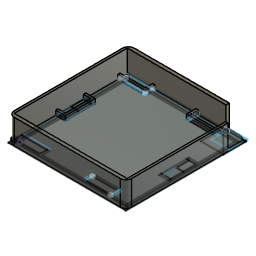
丐17磁悬浮验证底座 (Autodesk Fusion 360 design; units mm, degrees)
Autodesk Fusion 360 part; units mm, degrees
sketch "草图1" plane through (0, 0, 0) normal (0, 1, 0) x (1, 0, 0)
  line L0 (0, 0) -> (95.2, 0)
  line L1 (95.2, 0) -> (95.2, 95.4)
  line L2 (95.2, 95.4) -> (0, 95.4)
  line L3 (0, 95.4) -> (0, 0)
  line L4 (-1.5, 96.9) -> (96.7, 96.9)
  line L5 (96.7, 96.9) -> (96.7, -1.5)
  line L6 (96.7, -1.5) -> (-1.5, -1.5)
  line L7 (-1.5, -1.5) -> (-1.5, 96.9)
  line L8 (-2.5, 97.9) -> (97.7, 97.9)
  line L9 (97.7, 97.9) -> (97.7, -2.5)
  line L10 (97.7, -2.5) -> (-2.5, -2.5)
  line L11 (-2.5, -2.5) -> (-2.5, 97.9)
  line L12 (-4.5, 100.9) -> (99.7, 100.9)
  line L13 (99.7, 100.9) -> (99.7, -5.5)
  line L14 (99.7, -5.5) -> (-4.5, -5.5)
  line L15 (-4.5, -5.5) -> (-4.5, 100.9)
  line L16 (99.7, 100.9) -> (79.7, 100.9)
  line L17 (79.7, 100.9) -> (79.7, 80.9)
  line L18 (79.7, 80.9) -> (99.7, 80.9)
  line L19 (99.7, 80.9) -> (99.7, 100.9)
  line L20 (79.7, 100.9) -> (99.7, 80.9)
  dimension "d1" = 95.2
  dimension "d2" = 95.4
  dimension "d3" = 1.5
  dimension "d4" = 1.5
  dimension "d5" = 1.5
  dimension "d6" = 1.5
  dimension "d7" = 1
  dimension "d8" = 1
  dimension "d9" = 1
  dimension "d10" = 1
  dimension "d11" = 3
  dimension "d12" = 2
  dimension "d13" = 2
  dimension "d14" = 3
  dimension "d21" = 20
  dimension "d22" = 20
  constraint horizontal L0
  constraint vertical L1
  constraint horizontal L2
  constraint vertical L3
  constraint coincident L0.start L3.end
  constraint horizontal L4
  constraint vertical L5
  constraint horizontal L6
  constraint vertical L7
  constraint horizontal L8
  constraint vertical L9
  constraint horizontal L10
  constraint vertical L11
  constraint horizontal L12
  constraint vertical L13
  constraint horizontal L14
  constraint vertical L15
  constraint horizontal L16
  constraint vertical L17
  constraint horizontal L18
  constraint vertical L19
  measures "d1" distance of L0.start L0.end
  measures "d2" distance of L0.start L2.end
  measures "d3" distance of L2 L4
  measures "d4" distance of L1 L5
  measures "d5" distance of L0 L6
  measures "d6" distance of L3 L7
  measures "d7" distance of L4 L8
  measures "d8" distance of L5 L9
  measures "d9" distance of L6 L10
  measures "d10" distance of L7 L11
  measures "d11" distance of L8 L12
  measures "d12" distance of L11 L15
  measures "d13" distance of L9 L13
  measures "d14" distance of L10 L14
  measures "d21" distance of L12.end L16.end
  measures "d22" distance of L12.end L18.end
extrude "拉伸1" add sketch "草图1" along normal blind 2 contours L0 L1 L2 L3 L17 L18 | L0 L1 L2 L3 L4 L5 L6 L7 L17 L18 | L1 L2 L17 L18 L20 | L1 L5 L18 L20 | L2 L4 L17 L20 | L1 L2 L20 | L1 L2 L4 L5 L20 | L4 L5 L6 L7 L8 L9 L10 L11 L17 L18 | L5 L9 L18 L20 | L4 L8 L17 L20 | L4 L5 L8 L9 L20
extrude "拉伸2" add sketch "草图1" along normal blind 22 contours L8 L9 L10 L11 L12 L13 L14 L15 L17 L18 | L9 L18 L20 | L8 L17 L20 | L8 L9 L12 L13 L16 L19 L20
fillet "圆角1" radius 5 4 edges at (-4.5, 11, 5.5) (99.7, 11, 5.5) (-4.5, 11, -100.9) (99.7, 11, -100.9)
extrude "拉伸3" [suppressed]
fillet "圆角2" [suppressed]
sketch "草图2" plane through (0, 2, 0) normal (0, 1, 0) x (-1, 0, 0)
  line L0 (-97.7, -97.9) -> (2.5, -97.9)
  line L1 (2.5, -97.9) -> (2.5, 2.5)
  line L2 (2.5, 2.5) -> (-97.7, 2.5)
  line L3 (-97.7, 2.5) -> (-97.7, -97.9)
  line L4 (2.5, 2.5) -> (2.5, -20)
  line L5 (2.5, -20) -> (-5.5, -20)
  line L6 (-5.5, -20) -> (-5.5, -22)
  line L7 (-5.5, -22) -> (2.5, -22)
  line L8 (2.5, -22) -> (2.5, -20)
  line L9 (-5.5, -20) -> (-3.5, -20)
  line L10 (-3.5, -20) -> (-3.5, 2.5)
  line L11 (-3.5, 2.5) -> (-5.5, 2.5)
  line L12 (-5.5, 2.5) -> (-5.5, -20)
  line L13 (-97.7, 2.5) -> (-91.7, 2.5)
  line L14 (-91.7, 2.5) -> (-91.7, -20)
  line L15 (-91.7, -20) -> (-97.7, -20)
  line L16 (-97.7, -20) -> (-97.7, 2.5)
  line L17 (-97.7, -20) -> (-89.7, -20)
  line L18 (-89.7, -20) -> (-89.7, -23)
  line L19 (-89.7, -23) -> (-97.7, -23)
  line L20 (-97.7, -23) -> (-97.7, -20)
  line L21 (-89.7, -20) -> (-91.7, -20)
  line L22 (-91.7, -20) -> (-91.7, 2.5)
  line L23 (-91.7, 2.5) -> (-89.7, 2.5)
  line L24 (-89.7, 2.5) -> (-89.7, -20)
  line L25 (-91.7, -97.9) -> (-91.7, -75.4)
  line L26 (-91.7, -97.9) -> (-97.7, -97.9)
  line L27 (-97.7, -97.9) -> (-97.7, -75.4)
  line L28 (-97.7, -75.4) -> (-91.7, -75.4)
  line L29 (2.5, -97.9) -> (2.5, -75.4)
  line L30 (-3.5, -75.4) -> (2.5, -75.4)
  line L31 (-3.5, -97.9) -> (-3.5, -75.4)
  line L32 (2.5, -97.9) -> (-3.5, -97.9)
  line L33 (2.5, -75.4) -> (-5.5, -75.4)
  line L34 (-5.5, -75.4) -> (-5.5, -73.4)
  line L35 (-5.5, -73.4) -> (2.5, -73.4)
  line L36 (2.5, -73.4) -> (2.5, -75.4)
  line L37 (-5.5, -75.4) -> (-3.5, -75.4)
  line L38 (-3.5, -75.4) -> (-3.5, -97.9)
  line L39 (-3.5, -97.9) -> (-5.5, -97.9)
  line L40 (-5.5, -97.9) -> (-5.5, -75.4)
  line L41 (-97.7, -75.4) -> (-89.7, -75.4)
  line L42 (-89.7, -75.4) -> (-89.7, -73.4)
  line L43 (-89.7, -73.4) -> (-97.7, -73.4)
  line L44 (-97.7, -73.4) -> (-97.7, -75.4)
  line L45 (-89.7, -75.4) -> (-91.7, -75.4)
  line L46 (-91.7, -75.4) -> (-91.7, -97.9)
  line L47 (-91.7, -97.9) -> (-89.7, -97.9)
  line L48 (-89.7, -97.9) -> (-89.7, -75.4)
  line L49 (-47.6, -97.9) -> (-47.6, -91.9)
  line L50 (-47.6, -91.9) -> (-36.35, -91.9)
  line L51 (-47.6, -91.9) -> (-58.85, -91.9)
  line L52 (-36.35, -91.9) -> (-58.85, -91.9)
  line L53 (-58.85, -91.9) -> (-58.85, -97.9)
  line L54 (-58.85, -97.9) -> (-36.35, -97.9)
  line L55 (-36.35, -97.9) -> (-36.35, -91.9)
  line L56 (-47.6, 2.5) -> (-36.35, 2.5)
  line L57 (-36.35, -3.5) -> (-36.35, 2.5)
  line L58 (-58.85, -3.5) -> (-36.35, -3.5)
  line L59 (-36.35, 2.5) -> (-58.85, 2.5)
  line L60 (-58.85, 2.5) -> (-58.85, -3.5)
  line L61 (-36.35, -97.9) -> (-34.35, -97.9)
  line L62 (-34.35, -97.9) -> (-34.35, -89.9)
  line L63 (-34.35, -89.9) -> (-36.35, -89.9)
  line L64 (-36.35, -89.9) -> (-36.35, -97.9)
  line L65 (-36.35, -89.9) -> (-58.85, -89.9)
  line L66 (-58.85, -89.9) -> (-58.85, -91.9)
  line L67 (-58.85, -91.9) -> (-36.35, -91.9)
  line L68 (-36.35, -91.9) -> (-36.35, -89.9)
  line L69 (-58.85, -89.9) -> (-60.85, -89.9)
  line L70 (-60.85, -89.9) -> (-60.85, -97.9)
  line L71 (-60.85, -97.9) -> (-58.85, -97.9)
  line L72 (-58.85, -97.9) -> (-58.85, -89.9)
  line L73 (-36.35, 2.5) -> (-34.35, 2.5)
  line L74 (-34.35, 2.5) -> (-34.35, -5.5)
  line L75 (-34.35, -5.5) -> (-36.35, -5.5)
  line L76 (-36.35, -5.5) -> (-36.35, 2.5)
  line L77 (-58.85, 2.5) -> (-60.85, 2.5)
  line L78 (-60.85, 2.5) -> (-60.85, -5.5)
  line L79 (-60.85, -5.5) -> (-58.85, -5.5)
  line L80 (-58.85, -5.5) -> (-58.85, 2.5)
  line L81 (-36.35, -5.5) -> (-58.85, -5.5)
  line L82 (-58.85, -5.5) -> (-58.85, -3.5)
  line L83 (-58.85, -3.5) -> (-36.35, -3.5)
  line L84 (-36.35, -3.5) -> (-36.35, -5.5)
  dimension "d27" = 22.5
  dimension "d28" = 8
  dimension "d29" = 2
  dimension "d32" = 6
  dimension "d33" = 22.5
  dimension "d34" = 8
  dimension "d35" = 3
  dimension "d38" = 77.9
  dimension "d39" = 0
  dimension "d42" = 94.2
  dimension "d43" = 0
  dimension "d44" = 8
  dimension "d45" = 2
  dimension "d46" = 8
  dimension "d47" = 2
  dimension "d50" = 6
  dimension "d51" = 11.25
  dimension "d52" = 11.25
  dimension "d55" = 0
  dimension "d56" = 94.4
  dimension "d57" = 2
  dimension "d58" = 8
  dimension "d59" = 2
  dimension "d60" = 8
  dimension "d61" = 2
  dimension "d62" = 8
  dimension "d63" = 2
  dimension "d64" = 8
  constraint coincident L1.end L2.start
  constraint perpendicular L2 L4
  constraint vertical L6
  constraint horizontal L7
  constraint vertical L8
  constraint horizontal L9
  constraint vertical L10
  constraint horizontal L11
  constraint vertical L12
  constraint coincident L2 L10.end
  constraint horizontal L13
  constraint vertical L14
  constraint horizontal L15
  constraint vertical L16
  constraint coincident L2.end L3.start
  constraint horizontal L17
  constraint vertical L18
  constraint horizontal L19
  constraint vertical L20
  constraint horizontal L21
  constraint vertical L22
  constraint horizontal L23
  constraint vertical L24
  constraint horizontal L33
  constraint vertical L34
  constraint horizontal L35
  constraint vertical L36
  constraint horizontal L37
  constraint vertical L38
  constraint horizontal L39
  constraint vertical L40
  constraint horizontal L41
  constraint vertical L42
  constraint horizontal L43
  constraint vertical L44
  constraint horizontal L45
  constraint vertical L46
  constraint horizontal L47
  constraint vertical L48
  constraint midpoint L0 L49.start
  constraint perpendicular L0 L49
  constraint perpendicular L49 L50
  constraint perpendicular L49 L51
  constraint horizontal L52
  constraint vertical L53
  constraint horizontal L54
  constraint vertical L55
  constraint coincident L0 L53.end
  constraint horizontal L61
  constraint vertical L62
  constraint horizontal L63
  constraint vertical L64
  constraint horizontal L65
  constraint vertical L66
  constraint horizontal L67
  constraint vertical L68
  constraint horizontal L69
  constraint vertical L70
  constraint horizontal L71
  constraint vertical L72
  constraint horizontal L73
  constraint vertical L74
  constraint horizontal L75
  constraint vertical L76
  constraint horizontal L77
  constraint vertical L78
  constraint horizontal L79
  constraint vertical L80
  constraint horizontal L81
  constraint vertical L82
  constraint horizontal L83
  constraint vertical L84
  measures "d27" distance of L1.end L4.end
  measures "d28" distance of L4.end L5.end
  measures "d29" distance of L5.end L9.end
  measures "d32" distance of L2.end L13.end
  measures "d33" distance of L2.end L15.end
  measures "d34" distance of L15.end L17.end
  measures "d35" distance of L15.end L19.end
  measures "d44" distance of L29.end L33.end
  measures "d45" distance of L29.end L35.end
  measures "d46" distance of L27.end L41.end
  measures "d47" distance of L27.end L43.end
  measures "d50" distance of L49.start L49.end
  measures "d51" distance of L49.end L50.end
  measures "d52" distance of L49.end L51.end
  measures "d57" distance of L54.end L61.end
  measures "d58" distance of L54.end L63.end
  measures "d59" distance of L65.end L69.end
  measures "d60" distance of L65.end L53.end
  measures "d61" distance of L56.end L73.end
  measures "d62" distance of L56.end L75.end
  measures "d63" distance of L59.end L77.end
  measures "d64" distance of L59.end L79.end
extrude "拉伸4" [suppressed]
extrude "拉伸5" [suppressed]
extrude "拉伸6" [suppressed]
sketch "草图3" plane through (0, 2, 0) normal (0, 1, 0) x (-1, 0, 0)
  line L0 (2.5, 2.5) -> (-97.7, 2.5)
  line L1 (-97.7, 2.5) -> (-97.7, -97.9)
  line L2 (-97.7, -97.9) -> (2.5, -97.9)
  line L3 (2.5, -97.9) -> (2.5, 2.5)
  line L4 (2.5, 2.5) -> (-20, 2.5)
  line L5 (-20, 2.5) -> (-20, -4)
  line L6 (-20, -4) -> (2.5, -4)
  line L7 (2.5, -4) -> (2.5, 2.5)
  line L8 (2.5, -4) -> (-20, -4)
  line L9 (-20, -4) -> (-20, -6)
  line L10 (-20, -6) -> (2.5, -6)
  line L11 (2.5, -6) -> (2.5, -4)
  line L12 (-20, -6) -> (-22, -6)
  line L13 (-22, -6) -> (-22, 2.5)
  line L14 (-22, 2.5) -> (-20, 2.5)
  line L15 (-20, 2.5) -> (-20, -6)
  line L16 (-20, -91.4) -> (-20, -97.9)
  line L17 (-20, -97.9) -> (2.5, -97.9)
  line L18 (2.5, -97.9) -> (2.5, -91.4)
  line L19 (2.5, -91.4) -> (-20, -91.4)
  line L20 (2.5, -97.9) -> (-20, -97.9)
  line L21 (2.5, -91.4) -> (-20, -91.4)
  line L22 (-20, -91.4) -> (-20, -89.4)
  line L23 (-20, -89.4) -> (2.5, -89.4)
  line L24 (2.5, -89.4) -> (2.5, -91.4)
  line L25 (-20, -89.4) -> (-22, -89.4)
  line L26 (-22, -89.4) -> (-22, -97.9407)
  line L27 (-22, -97.9407) -> (-20, -97.9407)
  line L28 (-20, -97.9407) -> (-20, -89.4)
  line L29 (2.5, -47.7) -> (-4, -47.7)
  line L30 (-4, -47.7) -> (-4, -58.95)
  line L31 (-4, -58.95) -> (2.5, -58.95)
  line L32 (2.5, -58.95) -> (2.5, -47.7)
  line L33 (-4, -47.7) -> (2.5, -47.7)
  line L34 (2.5, -47.7) -> (2.5, -36.45)
  line L35 (2.5, -36.45) -> (-4, -36.45)
  line L36 (-4, -36.45) -> (-4, -47.7)
  line L37 (-97.7, -36.45) -> (-97.7, -47.7)
  line L38 (-91.2, -47.7) -> (-91.2, -36.45)
  line L39 (-97.7, -47.7) -> (-97.7, -58.95)
  line L40 (-91.2, -58.95) -> (-91.2, -47.7)
  line L41 (-91.2, -36.45) -> (-97.7, -36.45)
  line L42 (-91.2, -47.7) -> (-97.7, -47.7)
  line L43 (-97.7, -47.7) -> (-91.2, -47.7)
  line L44 (-97.7, -58.95) -> (-91.2, -58.95)
  line L45 (2.5, -36.45) -> (-6, -36.45)
  line L46 (-6, -36.45) -> (-6, -34.45)
  line L47 (-6, -34.45) -> (2.5, -34.45)
  line L48 (2.5, -34.45) -> (2.5, -36.45)
  line L49 (-4, -58.95) -> (-6, -58.95)
  line L50 (-6, -58.95) -> (-6, -36.45)
  line L51 (-6, -36.45) -> (-4, -36.45)
  line L52 (-4, -36.45) -> (-4, -58.95)
  line L53 (-6, -58.95) -> (2.5, -58.95)
  line L54 (2.5, -58.95) -> (2.5, -60.95)
  line L55 (2.5, -60.95) -> (-6, -60.95)
  line L56 (-6, -60.95) -> (-6, -58.95)
  line L57 (-97.7, -36.45) -> (-89.2, -36.45)
  line L58 (-89.2, -36.45) -> (-89.2, -34.45)
  line L59 (-89.2, -34.45) -> (-97.7, -34.45)
  line L60 (-97.7, -34.45) -> (-97.7, -36.45)
  line L61 (-89.2, -36.45) -> (-91.2, -36.45)
  line L62 (-91.2, -36.45) -> (-91.2, -58.95)
  line L63 (-91.2, -58.95) -> (-89.2, -58.95)
  line L64 (-89.2, -58.95) -> (-89.2, -36.45)
  line L65 (-89.2, -58.95) -> (-97.7, -58.95)
  line L66 (-97.7, -58.95) -> (-97.7, -60.95)
  line L67 (-97.7, -60.95) -> (-89.2, -60.95)
  line L68 (-89.2, -60.95) -> (-89.2, -58.95)
  line L69 (-101, -101) -> (-85, -101)
  line L70 (-85, -101) -> (-85, -85)
  line L71 (-85, -85) -> (-101, -85)
  line L72 (-101, -85) -> (-101, -101)
  line L73 (-85, -97.9) -> (-83, -97.9)
  line L74 (-83, -97.9) -> (-83, -89.4)
  line L75 (-83, -89.4) -> (-85, -89.4)
  line L76 (-85, -89.4) -> (-85, -97.9)
  line L77 (-83, -97.9) -> (-60.5, -97.9)
  line L78 (-60.5, -97.9) -> (-60.5, -91.4)
  line L79 (-60.5, -91.4) -> (-83, -91.4)
  line L80 (-83, -91.4) -> (-83, -97.9)
  line L81 (-83, -89.4) -> (-60.5, -89.4)
  line L82 (-60.5, -89.4) -> (-60.5, -91.4)
  line L83 (-60.5, -91.4) -> (-83, -91.4)
  line L84 (-83, -91.4) -> (-83, -89.4)
  line L85 (-60.5, -89.4) -> (-58.5, -89.4)
  line L86 (-58.5, -89.4) -> (-58.5, -97.9)
  line L87 (-58.5, -97.9) -> (-60.5, -97.9)
  line L88 (-60.5, -97.9) -> (-60.5, -89.4)
  line L89 (-60.5, 2.5) -> (-83, 2.5)
  line L90 (-60.5, 2.5) -> (-83, 2.5)
  line L91 (-83, -4) -> (-60.5, -4)
  line L92 (-60.5, -4) -> (-60.5, 2.5)
  line L93 (-83, 2.5) -> (-83, -4)
  line L94 (-60.5, 2.5) -> (-58.5, 2.5)
  line L95 (-58.5, 2.5) -> (-58.5, -6)
  line L96 (-58.5, -6) -> (-60.5, -6)
  line L97 (-60.5, -6) -> (-60.5, 2.5)
  line L98 (-60.5, -6) -> (-83, -6)
  line L99 (-83, -6) -> (-83, -4)
  line L100 (-83, -4) -> (-60.5, -4)
  line L101 (-60.5, -4) -> (-60.5, -6)
  line L102 (-83, -6) -> (-85, -6)
  line L103 (-85, -6) -> (-85, 2.5)
  line L104 (-85, 2.5) -> (-83, 2.5)
  line L105 (-83, 2.5) -> (-83, -6)
  point P0 (-20, -91.4)
  point P1 (2.5, -91.4)
  point P2 (0, -93.9)
  point P3 (-60.5, -4)
  dimension "d67" = 22.5
  dimension "d68" = 6.5
  dimension "d69" = 22.5
  dimension "d70" = 2
  dimension "d79" = 2
  dimension "d80" = 2
  dimension "d84" = 6.5
  dimension "d85" = 11.25
  dimension "d86" = 11.25
  dimension "d89" = -93.7
  dimension "d90" = 0
  dimension "d91" = 8.5
  dimension "d92" = 2
  dimension "d93" = 2
  dimension "d94" = 8.5
  dimension "d95" = 2
  dimension "d96" = 2
  dimension "d101" = 2
  dimension "d102" = 8.5
  dimension "d103" = 22.5
  dimension "d104" = 6.5
  dimension "d105" = 2
  dimension "d108" = -93.9
  dimension "d109" = 0
  dimension "d110" = 2
  dimension "d111" = 8.5
  dimension "d112" = 2
  constraint horizontal L4
  constraint vertical L5
  constraint horizontal L6
  constraint vertical L7
  constraint coincident L0.start L3.end
  constraint horizontal L8
  constraint vertical L9
  constraint horizontal L10
  constraint vertical L11
  constraint horizontal L12
  constraint vertical L13
  constraint horizontal L14
  constraint vertical L15
  constraint horizontal L21
  constraint vertical L22
  constraint horizontal L23
  constraint vertical L24
  constraint horizontal L25
  constraint vertical L26
  constraint horizontal L27
  constraint vertical L28
  constraint horizontal L29
  constraint vertical L30
  constraint horizontal L31
  constraint vertical L32
  constraint midpoint L3 L29.start
  constraint horizontal L33
  constraint vertical L34
  constraint horizontal L35
  constraint vertical L36
  constraint horizontal L45
  constraint vertical L46
  constraint horizontal L47
  constraint vertical L48
  constraint horizontal L49
  constraint vertical L50
  constraint horizontal L51
  constraint vertical L52
  constraint horizontal L53
  constraint vertical L54
  constraint horizontal L55
  constraint vertical L56
  constraint horizontal L57
  constraint vertical L58
  constraint horizontal L59
  constraint vertical L60
  constraint horizontal L61
  constraint vertical L62
  constraint horizontal L63
  constraint vertical L64
  constraint horizontal L65
  constraint vertical L66
  constraint horizontal L67
  constraint vertical L68
  constraint horizontal L69
  constraint vertical L70
  constraint horizontal L71
  constraint vertical L72
  constraint horizontal L73
  constraint vertical L74
  constraint horizontal L75
  constraint vertical L76
  constraint coincident L70 L73.start
  constraint coincident L2 L73.start
  constraint horizontal L77
  constraint vertical L78
  constraint horizontal L79
  constraint vertical L80
  constraint horizontal L81
  constraint vertical L82
  constraint horizontal L83
  constraint vertical L84
  constraint horizontal L85
  constraint vertical L86
  constraint horizontal L87
  constraint vertical L88
  constraint coincident L2 L86.end
  constraint horizontal L94
  constraint vertical L95
  constraint horizontal L96
  constraint vertical L97
  constraint horizontal L98
  constraint vertical L99
  constraint horizontal L100
  constraint vertical L101
  constraint horizontal L102
  constraint vertical L103
  constraint horizontal L104
  constraint vertical L105
  measures "d67" distance of L0.start L4.end
  measures "d68" distance of L0.start L6.end
  measures "d69" distance of L6.end L5.end
  measures "d70" distance of L9.end L12.end
  measures "d79" distance of P1 L23.end
  measures "d80" distance of L22.end L25.end
  measures "d84" distance of L29.start L29.end
  measures "d85" distance of L29.start L31.end
  measures "d86" distance of L29.end L35.end
  measures "d91" distance of L34.end L45.end
  measures "d92" distance of L34.end L47.end
  measures "d93" distance of L49.end L55.end
  measures "d94" distance of L37.start L57.end
  measures "d95" distance of L37.start L59.end
  measures "d96" distance of L63.end L67.end
  measures "d101" distance of L73.start L73.end
  measures "d102" distance of L73.start L75.end
  measures "d103" distance of L73.end L77.end
  measures "d104" distance of L73.end L79.end
  measures "d105" distance of L81.end L85.end
  measures "d110" distance of L89.start L94.end
  measures "d111" distance of L89.start L96.end
  measures "d112" distance of L98.end L102.end
extrude "拉伸8" cut sketch "草图3" along normal blind 24 contours L1 L2 L69 L70 L71 L72
extrude "拉伸9" add sketch "草图3" along normal blind 4 contours L0 L5 L9 L12 L13 L14 L15 | L3 L6 L8 L9 L10 L11 L15 | L0 L92 L94 L95 L96 L97 L101 | L3 L35 L45 L46 L47 L48 L51 | L0 L93 L99 L102 L103 L104 L105 | L91 L97 L98 L99 L100 L101 L105 | L30 L36 L45 L49 L50 L51 L52 L53 | L3 L31 L49 L53 L54 L55 L56 | L1 L41 L57 L58 L59 L60 L61 | L3 L19 L21 L22 L23 L24 L28 | L2 L16 L22 L25 L26 L28 | L38 L40 L57 L61 L62 L63 L64 L65 | L1 L44 L63 L65 L66 L67 L68 | L2 L78 L82 L85 L86 L87 L88 | L2 L70 L73 L74 L75 L76 L80 L84 | L74 L79 L81 L82 L83 L84 L88
